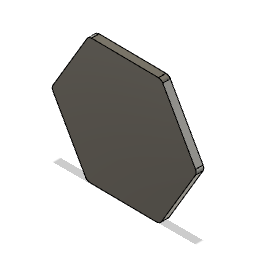
medallion 1 basic v1 (Autodesk Fusion 360 design; units mm, degrees)
Autodesk Fusion 360 part; units mm, degrees
note: some values were not read from the file. Set by a fixed rule: which sketch regions a step uses.
sketch "Sketch1" plane through (0, 0, 0) normal (0, 0, 1) x (1, 0, 0)
  line L0 (13.5687, 24.844) -> (-12.9876, 25.1527)
  line L1 (-14.7311, 24.1729) -> (-28.2766, 1.3288)
  line L2 (-28.2999, -0.6711) -> (-15.2891, -23.8239)
  line L3 (-13.5687, -24.844) -> (12.9876, -25.1527)
  line L4 (14.7311, -24.1729) -> (28.2766, -1.3288)
  line L5 (28.2999, 0.6711) -> (15.2891, 23.8239)
  arc A0 (-12.9876, 25.1527) -> (-14.7311, 24.1729) centre (-13.0108, 23.1528) ccw
  arc A1 (15.2891, 23.8239) -> (13.5687, 24.844) centre (13.5455, 22.8441) ccw
  arc A2 (28.2766, -1.3288) -> (28.2999, 0.6711) centre (26.5563, -0.3087) ccw
  arc A3 (12.9876, -25.1527) -> (14.7311, -24.1729) centre (13.0108, -23.1528) ccw
  arc A4 (-15.2891, -23.8239) -> (-13.5687, -24.844) centre (-13.5455, -22.8441) ccw
  arc A5 (-28.2766, 1.3288) -> (-28.2999, -0.6711) centre (-26.5563, 0.3087) ccw
  point P0 (-12.5, 7.2169)
  dimension "d1" = 25
  dimension "d7" = 2
  dimension "d8" = 2
  dimension "d9" = 2
  dimension "d10" = 2
  dimension "d11" = 2
  dimension "d12" = 2
  constraint tangent L0 A0
  constraint tangent L1 A0
  constraint tangent L0 A1
  constraint tangent L5 A1
  constraint tangent L4 A2
  constraint tangent L5 A2
  constraint tangent L3 A3
  constraint tangent L4 A3
  constraint tangent L2 A4
  constraint tangent L3 A4
  constraint tangent L1 A5
  constraint tangent L2 A5
  measures "d1" distance of origin L5
  measures "d7" radius of A0
  measures "d8" radius of A1
  measures "d9" radius of A2
  measures "d10" radius of A3
  measures "d11" radius of A4
  measures "d12" radius of A5
extrude "Extrude1" add sketch "Sketch1" along normal blind 3
